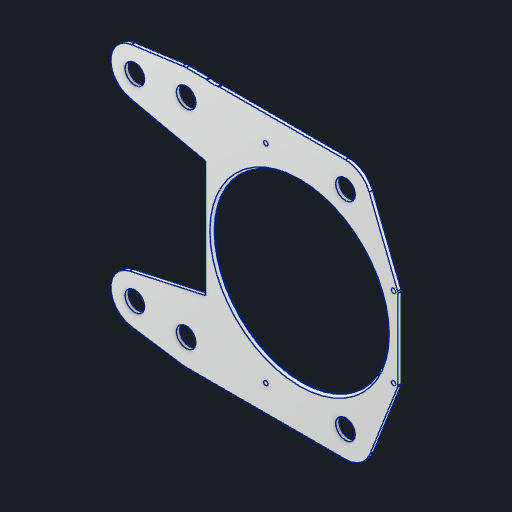
# Autodesk Inventor part: OUTK_002_ShotPlateReceptacle
Saved by Autodesk Inventor 2024.2 (Build 282272000, 272)
## iProperties
Created: 2024-11-24
Part Number: OUTK_002_ShotPlateReceptacle
Material: Aluminum 6061
Document SubType Name: Modeling
Designer: Bryan
Density: 2.7 g/cm^3
Appearance: Aluminum - Flat
Mass: 837.54 g
Surface Area: 1450.99 cm^2
Volume: 310.2 cm^3
Author: Bryan
Autodesk Inventor part; units mm, degrees
ref_plane "YZ Plane" through (0, 0, 0) normal (1, 0, 0) x (0, 1, 0)
ref_plane "XZ Plane" through (0, 0, 0) normal (0, 1, 0) x (-1, 0, 0)
ref_plane "XY Plane" through (0, 0, 0) normal (0, 0, 1) x (1, 0, 0)
sketch "Sketch1" plane through (0, 0, 0) normal (0, 0, 1) x (1, 0, 0)
  circle A0 centre (0, 142.875) radius 63.5 construction
  circle A1 centre (0, 142.875) radius 25.4 construction
  circle A2 centre (0, -142.875) radius 25.4 construction
  circle A3 centre (0, -142.875) radius 63.5 construction
  line L0 (0, 79.375) -> (0, 79.375) construction
  line L1 (0, -79.375) -> (0, -79.375) construction
  line L2 (0, 0) -> (229.6782, 0) construction
  line L3 (0, 142.875) -> (305.8782, 142.875) construction
  line L4 (305.8782, 142.875) -> (305.8782, -142.875) construction
  line L5 (305.8782, -142.875) -> (0, -142.875) construction
  circle A4 centre (229.6782, 0) radius 127 construction
  circle A5 centre (0, 142.875) radius 14.2875
  circle A6 centre (0, -142.875) radius 14.2875
  circle A7 centre (0, 142.875) radius 34.925 construction
  circle A8 centre (0, -142.875) radius 34.925 construction
  circle A9 centre (74.585, -150.8125) radius 22.225 construction
  circle A10 centre (74.585, -150.8125) radius 33.3375 construction
  circle A11 centre (74.585, -150.8125) radius 11.1125 construction
  line L6 (74.585, -139.7) -> (74.585, -128.5875) construction
  line L7 (74.585, -117.475) -> (74.585, -128.5875) construction
  circle A12 centre (305.8782, -150.8125) radius 33.3375 construction
  circle A13 centre (305.8782, -150.8125) radius 14.2875
  circle A14 centre (375.7282, 58.0572) radius 6.35 construction
  circle A15 centre (375.7282, -58.0572) radius 6.35 construction
  line L8 (305.8782, 150.8125) -> (375.7282, 58.0572) construction
  line L9 (375.7282, 58.0572) -> (375.7282, -58.0572) construction
  line L10 (375.7282, -58.0572) -> (305.8782, -150.8125) construction
  line L11 (-117.6668, 84.5312) -> (102.6782, 84.5312) construction
  line L12 (102.6782, 84.5312) -> (102.6782, -84.5312) construction
  line L13 (102.6782, -84.5312) -> (-117.6668, -84.5312) construction
  line L14 (-117.6668, -84.5312) -> (-117.6668, 84.5312) construction
  line L15 (0, 142.875) -> (0, 84.5312) construction
  line L16 (0, -84.5312) -> (0, -142.875) construction
  circle A16 centre (74.585, -150.8125) radius 14.2875
  line L17 (74.585, -117.475) -> (305.8782, -117.475) construction
  circle A17 centre (74.585, 0) radius 127 construction
  circle A18 centre (0, 0) radius 127 construction
  circle A19 centre (0, 142.875) radius 6.35 construction
  circle A20 centre (74.585, 150.8125) radius 33.3375 construction
  circle A21 centre (305.8782, 150.8125) radius 33.3375 construction
  circle A22 centre (305.8782, 150.8125) radius 14.2875
  circle A23 centre (74.585, 150.8125) radius 14.2875
  circle A24 centre (74.585, 150.8125) radius 37.1475 construction
  circle A25 centre (305.8782, 150.8125) radius 37.1475 construction
  circle A26 centre (305.8782, -150.8125) radius 38.1 construction
  circle A27 centre (74.585, -150.8125) radius 38.1 construction
  line L18 (-4.7233, 177.4791) -> (69.5611, 187.6187)
  line L19 (74.585, 187.96) -> (305.8782, 187.96)
  line L20 (340.4169, 164.488) -> (381.6323, 60.3949)
  line L21 (382.0782, 58.0572) -> (382.0782, -58.0572)
  line L22 (68.953, -188.4939) -> (-5.1627, -177.4163)
  line L23 (221.4945, -245.7989) -> (238.8691, -293.5353) construction
  line L24 (238.8691, -293.5353) -> (382.0782, -241.4114) construction
  line L25 (382.0782, -241.4114) -> (364.7036, -193.675) construction
  line L26 (364.7036, -193.675) -> (221.4945, -245.7989) construction
  line L27 (-7.5024, -108.7653) -> (102.6782, -84.5312)
  line L28 (-7.5024, 108.7653) -> (102.6782, 84.5312)
  line L29 (102.6782, 84.5312) -> (102.6782, -84.5312)
  circle A28 centre (239.2032, 0) radius 127
  line L30 (102.6782, 0) -> (112.2032, 0)
  line L31 (375.7282, 0) -> (366.2032, 0)
  circle A29 centre (221.4945, -245.7989) radius 3.2512 construction
  circle A30 centre (269.2308, -228.4242) radius 3.2512 construction
  circle A31 centre (316.9672, -211.0496) radius 3.2512 construction
  circle A32 centre (364.7036, -193.675) radius 3.2512 construction
  circle A33 centre (238.8691, -293.5353) radius 3.2512 construction
  circle A34 centre (286.6055, -276.1606) radius 3.2512 construction
  circle A35 centre (334.3418, -258.786) radius 3.2512 construction
  circle A36 centre (382.0782, -241.4114) radius 3.2512 construction
  line L32 (74.585, -188.9125) -> (305.8782, -188.9125)
  line L33 (381.652, -60.3445) -> (341.4207, -164.5364)
  arc A37 (-4.7233, 177.4791) -> (-7.5024, 108.7653) centre (0, 142.875) ccw
  arc A38 (74.585, 187.96) -> (69.5611, 187.6187) centre (74.585, 150.8125) ccw
  arc A39 (340.4169, 164.488) -> (305.8782, 187.96) centre (305.8782, 150.8125) ccw
  arc A40 (382.0782, 58.0572) -> (381.6323, 60.3949) centre (375.7282, 58.0572) ccw
  arc A41 (381.652, -60.3445) -> (382.0782, -58.0572) centre (375.7282, -58.0572) ccw
  arc A42 (305.8782, -188.9125) -> (341.4207, -164.5364) centre (305.8782, -150.8125) ccw
  arc A43 (68.953, -188.4939) -> (74.585, -188.9125) centre (74.585, -150.8125) ccw
  arc A44 (-7.5024, -108.7653) -> (-5.1627, -177.4163) centre (0, -142.875) ccw
  circle A45 centre (375.7282, 58.0572) radius 3.2512
  circle A46 centre (375.7282, -58.0572) radius 3.2512
  circle A47 centre (190.2316, 150.8125) radius 3.2512
  line L34 (74.585, 150.8125) -> (190.2316, 150.8125) construction
  line L35 (190.2316, 150.8125) -> (305.8782, 150.8125) construction
  circle A48 centre (190.2316, -150.8125) radius 3.2512
  point P0 (0, 117.475)
  point P1 (0, -117.475)
  point P2 (305.8782, 0)
  point P3 (229.6782, -127)
  point P4 (229.6782, -127)
  point P5 (356.6782, 0)
  point P6 (0, 127)
  point P7 (0, 117.475)
  point P8 (0, 136.525)
  dimension "d1" = 50.8
  dimension "d16" = 44.45
  dimension "d20" = 22.225
  dimension "d33" = 12.7
  dimension "d0" = 127
  dimension "d3" = 285.75
  dimension "d4" = 254
  dimension "d6" = 158.75
  dimension "d7" = 234.95
  dimension "d11" = 28.575
  dimension "d12" = 28.575
  dimension "d13" = 69.85
  dimension "d14" = 69.85
  dimension "d19" = 76.2
  dimension "d24" = 28.575
  dimension "d26" = 12.7
  dimension "d27" = 12.7
  dimension "d28" = 19.05
  dimension "d29" = 220.345
  dimension "d30" = 169.0624
  dimension "d31" = 9.525
  dimension "d32" = 75.0062
  dimension "d34" = 9.525
  dimension "d35" = 19.05
  dimension "d37" = 3.81
  dimension "d38" = 3.81
  dimension "d39" = 4.7625
  dimension "d40" = 4.7625
  dimension "d43" = 20
  dimension "d44" = 6.5024
  dimension "d47" = 50.8
  dimension "d50" = 50.8
  dimension "d53" = 50.8
  dimension "d56" = 6.5024
  dimension "d57" = 6.5024
  dimension "d58" = 6.5024
  dimension "d108" = 231.2932
  constraints: 72 end point, 41 centre point, 41 point on circle, 24 tangent, 21 coincident, 16 vertical alignment, 11 horizontal, 7 perpendicular, 7 point on line, 6 concentric, 6 equal length, 6 symmetric about line, 4 equal radius, 4 vertical, 3 horizontal alignment, 3 midpoint, 2 parallel, 41 other
  measures "d0" diameter of A0
  measures "d3" distance between parallel lines of L5 L3
  measures "d4" diameter of A4
  measures "d6" distance of L1.start L0.start
  measures "d7" distance of point (0, -117.475) point (0, 117.475)
  measures "d11" diameter of A5
  measures "d12" diameter of A6
  measures "d13" diameter of A7
  measures "d14" diameter of A8
  measures "d19" distance of point (305.878, 0) L2.end
  measures "d24" diameter of A13
  measures "d26" diameter of A14
  measures "d27" diameter of A15
  measures "d28" distance from line of L9 point (356.678, 0)
  measures "d29" distance of L12.end L13.end
  measures "d30" distance of L11.end L12.end
  measures "d31" distance from line of L17 A4.start
  measures "d32" distance of point (74.585, -150.812) point (0, -142.875)
  measures "d34" distance of point (0, 117.475) point (0, 127)
  measures "d35" distance of point (0, 117.475) point (0, 136.525)
  measures "d37" radial gap between concentric circles of A20 A24
  measures "d38" radial gap between concentric circles of A21 A25
  measures "d43" angle of L26 L5
  measures "d44" diameter of A29
  measures "d47" distance of A29.centre A30.centre
  measures "d50" distance of A29.centre A33.centre
  measures "d53" distance from line of L25.end L5
  measures "d56" diameter of A45
  measures "d57" diameter of A46
  measures "d58" diameter of A47
  measures "d108" distance of L8.start A23.centre
extrude "Extrusion1" add sketch "Sketch1" along normal mid plane 4.7625
sketch "Sketch2" plane through (0, 0, -2.3813) normal (0, 0, -1) x (-1, 0, 0)
  line L0 (7.5024, -108.7653) -> (-102.6782, -84.5312) projected
  line L1 (-102.6782, -84.5312) -> (-102.6782, 84.5312) projected
  line L2 (-102.6782, 84.5312) -> (7.5024, 108.7653) projected
  arc A0 (7.5024, 108.7653) -> (4.7233, 177.4791) centre (0, 142.875) ccw projected
  line L3 (4.7233, 177.4791) -> (-69.5611, 187.6187) projected
  arc A1 (-69.5611, 187.6187) -> (-74.585, 187.96) centre (-74.585, 150.8125) ccw projected
  line L4 (-74.585, 187.96) -> (-305.8782, 187.96) projected
  arc A2 (-305.8782, 187.96) -> (-340.4169, 164.488) centre (-305.8782, 150.8125) ccw projected
  line L5 (-340.4169, 164.488) -> (-381.6323, 60.3949) projected
  arc A3 (-381.6323, 60.3949) -> (-382.0782, 58.0572) centre (-375.7282, 58.0572) ccw projected
  line L6 (-382.0782, 58.0572) -> (-382.0782, -58.0572) projected
  arc A4 (-382.0782, -58.0572) -> (-381.652, -60.3445) centre (-375.7282, -58.0572) ccw projected
  line L7 (-381.652, -60.3445) -> (-341.4207, -164.5364) projected
  arc A5 (-341.4207, -164.5364) -> (-305.8782, -188.9125) centre (-305.8782, -150.8125) ccw projected
  line L8 (-305.8782, -188.9125) -> (-74.585, -188.9125) projected
  arc A6 (-74.585, -188.9125) -> (-68.953, -188.4939) centre (-74.585, -150.8125) ccw projected
  line L9 (-68.953, -188.4939) -> (5.1627, -177.4163) projected
  arc A7 (5.1627, -177.4163) -> (7.5024, -108.7653) centre (0, -142.875) ccw projected
  circle A8 centre (-239.2032, 0) radius 127 projected
  circle A9 centre (-74.585, -150.8125) radius 14.2875 projected
  circle A10 centre (-74.585, 150.8125) radius 14.2875 projected
  circle A11 centre (-190.2316, 150.8125) radius 3.2512 projected
  circle A12 centre (-190.2316, -150.8125) radius 3.2512 projected
  circle A13 centre (-375.7282, -58.0572) radius 3.2512 projected
  circle A14 centre (-375.7282, 58.0572) radius 3.2512 projected
  circle A15 centre (-305.8782, 150.8125) radius 14.2875 projected
  circle A16 centre (-305.8782, -150.8125) radius 14.2875 projected
  circle A17 centre (0, -142.875) radius 14.2875 projected
  circle A18 centre (0, 142.875) radius 14.2875 projected
  line L10 (-107.4407, -88.36) -> (6.4793, -113.4166)
  arc A19 (4.4587, -172.7061) -> (6.4793, -113.4166) centre (0, -142.875) ccw
  line L11 (4.4587, -172.7061) -> (-69.657, -183.7838)
  arc A20 (-74.585, -184.15) -> (-69.657, -183.7838) centre (-74.585, -150.8125) ccw
  line L12 (-74.585, -184.15) -> (-305.8782, -184.15)
  arc A21 (-336.9779, -162.8209) -> (-305.8782, -184.15) centre (-305.8782, -150.8125) ccw
  line L13 (-336.9779, -162.8209) -> (-377.2092, -58.6291)
  arc A22 (-377.3157, -58.0572) -> (-377.2092, -58.6291) centre (-375.7282, -58.0572) ccw
  line L14 (-377.3157, -58.0572) -> (-377.3157, 58.0572)
  arc A23 (-377.2042, 58.6416) -> (-377.3157, 58.0572) centre (-375.7282, 58.0572) ccw
  line L15 (-377.2042, 58.6416) -> (-335.9888, 162.7347)
  arc A24 (-305.8782, 183.1975) -> (-335.9888, 162.7347) centre (-305.8782, 150.8125) ccw
  line L16 (-305.8782, 183.1975) -> (-74.585, 183.1975)
  arc A25 (-70.2052, 182.9) -> (-74.585, 183.1975) centre (-74.585, 150.8125) ccw
  line L17 (-70.2052, 182.9) -> (4.0793, 172.7604)
  arc A26 (6.4793, 113.4166) -> (4.0793, 172.7604) centre (0, 142.875) ccw
  line L18 (6.4793, 113.4166) -> (-107.4407, 88.36)
  line L19 (-107.4407, 88.36) -> (-107.4407, -88.36)
  circle A27 centre (-239.2032, 0) radius 133.35
  circle A28 centre (-74.585, 150.8125) radius 19.05
  circle A29 centre (0, 142.875) radius 19.05
  circle A30 centre (-190.2316, 150.8125) radius 8.0137
  circle A31 centre (-305.8782, 150.8125) radius 19.05
  circle A32 centre (-375.7282, 58.0572) radius 8.0137
  circle A33 centre (-375.7282, -58.0572) radius 8.0137
  circle A34 centre (-305.8782, -150.8125) radius 19.05
  circle A35 centre (-190.2316, -150.8125) radius 8.0137
  circle A36 centre (-74.585, -150.8125) radius 19.05
  circle A37 centre (0, -142.875) radius 19.05
  line L20 (0, -142.875) -> (-74.585, -150.8125)
  line L21 (-74.585, -150.8125) -> (-71.7613, -188.8077)
  line L22 (-74.585, -150.8125) -> (-102.6782, -84.5312)
  line L23 (-74.585, -150.8125) -> (-190.2316, -150.8125)
  line L24 (-190.2316, -150.8125) -> (-190.2316, -188.9125)
  line L25 (-190.2316, -150.8125) -> (-305.8782, -150.8125)
  line L26 (-305.8782, -150.8125) -> (-327.4274, -182.233)
  line L27 (-102.6782, -84.5312) -> (-239.2032, 0)
  line L28 (-239.2032, 0) -> (-190.2316, -150.8125)
  line L29 (-305.8782, -150.8125) -> (-239.2032, 0)
  line L30 (-239.2032, 0) -> (-375.7282, -58.0572)
  line L31 (-239.2032, 0) -> (-375.7282, 58.0572)
  line L32 (-375.7282, 58.0572) -> (-305.8782, 150.8125)
  line L33 (-305.8782, 150.8125) -> (-190.2316, 150.8125)
  line L34 (-190.2316, 150.8125) -> (-74.585, 150.8125)
  line L35 (-74.585, 150.8125) -> (0, 142.875)
  line L36 (-102.6782, -84.5312) -> (-190.2316, -150.8125)
  line L37 (-305.8782, -150.8125) -> (-375.7282, -58.0572)
  line L38 (-102.6782, 84.5312) -> (-74.585, 150.8125)
  line L39 (-102.6782, 84.5312) -> (-190.2316, 150.8125)
  line L40 (-102.6782, 84.5312) -> (-239.2032, 0)
  line L41 (-239.2032, 0) -> (-190.2316, 150.8125)
  line L42 (-239.2032, 0) -> (-305.8782, 150.8125)
  line L43 (-4.7625, -138.5924) -> (-75.089, -146.0767)
  line L44 (-68.936, -151.9364) -> (-99.5574, -79.6902)
  line L45 (0, -142.875) -> (0, -111.9915)
  line L46 (-4.7625, -110.944) -> (-4.7625, -138.5924)
  line L47 (0, 142.875) -> (0, 111.9915)
  line L48 (-99.5574, 79.6902) -> (-68.936, 151.9364)
  line L49 (-108.3272, 83.4073) -> (-77.7058, 155.6535)
  line L50 (-190.2316, 146.05) -> (-74.585, 146.05)
  line L51 (-98.0687, 87.0149) -> (-189.092, 155.923)
  line L52 (-105.1853, 88.5804) -> (-241.7103, 4.0492)
  line L53 (-103.8179, 79.4207) -> (-194.8411, 148.3288)
  line L54 (-235.7016, -4.6369) -> (-184.6739, 152.5077)
  line L55 (-244.761, -1.6952) -> (-193.7332, 155.4494)
  line L56 (-305.8782, 146.05) -> (-190.2316, 146.05)
  line L57 (-233.5511, -1.0064) -> (-302.8187, 155.6703)
  line L58 (-242.2627, -4.8578) -> (-311.5303, 151.8189)
  line L59 (-300.8665, 149.5508) -> (-368.2605, 60.0568)
  line L60 (-368.2605, 60.0568) -> (-236.9729, 4.2268)
  line L61 (-240.7003, -4.5386) -> (-383.1959, 56.0576)
  line L62 (-383.1959, 56.0576) -> (-308.4753, 155.2807)
  line L63 (-240.7003, 4.5386) -> (-383.1959, -56.0576)
  line L64 (-383.1959, -56.0576) -> (-308.4753, -155.2807)
  line L65 (-236.9729, -4.2268) -> (-368.2605, -60.0568)
  line L66 (-368.2605, -60.0568) -> (-300.8665, -149.5508)
  line L67 (-311.5303, -151.8189) -> (-242.2627, 4.8578)
  line L68 (-244.761, 1.6952) -> (-193.7332, -155.4494)
  line L69 (-235.7016, 4.6369) -> (-184.6739, -152.5077)
  line L70 (-302.8187, -155.6703) -> (-233.5511, 1.0064)
  line L71 (-105.1853, -88.5804) -> (-241.7103, -4.0492)
  line L72 (-100.1711, -80.482) -> (-236.6961, 4.0492)
  line L73 (-100.1711, 80.482) -> (-236.6961, -4.0492)
  line L74 (-77.7058, -155.6535) -> (-108.3272, -83.4073)
  line L75 (-105.5995, -80.7694) -> (-196.6227, -149.6775)
  line L76 (-98.0687, -87.0149) -> (-189.092, -155.923)
  line L77 (-74.585, -146.05) -> (-190.2316, -146.05)
  line L78 (-190.2316, -146.05) -> (-305.8782, -146.05)
  line L79 (-75.089, 146.0767) -> (-4.7625, 138.5924)
  line L80 (-4.7625, 138.5924) -> (-4.7625, 110.944)
  arc A38 (-377.3157, -6.35) -> (-372.4074, -6.2352) centre (-374.8602, -6.35) ccw
  arc A39 (-372.4074, 6.2352) -> (-377.3157, 6.35) centre (-374.8602, 6.35) ccw
  line L81 (-239.2032, 0) -> (-366.2032, 0)
  point P0 (0, 0)
  dimension "d59" = 4.7625
  dimension "d60" = 6.35
  dimension "d61" = 4.7625
  dimension "d62" = 4.7625
  dimension "d63" = 4.7625
  dimension "d64" = 4.7625
  dimension "d65" = 4.7625
  dimension "d66" = 4.7625
  dimension "d67" = 4.7625
  dimension "d68" = 4.7625
  dimension "d69" = 4.7625
  dimension "d70" = 4.7625
  dimension "d71" = 4.7625
  dimension "d72" = 4.7625
  dimension "d73" = 4.7625
  dimension "d75" = 4.7625
  dimension "d76" = 4.7625
  dimension "d77" = 4.7625
  dimension "d78" = 4.7625
  dimension "d79" = 4.7625
  dimension "d80" = 4.7625
  dimension "d81" = 4.7625
  dimension "d82" = 4.7625
  dimension "d83" = 4.7625
  dimension "d84" = 4.7625
  dimension "d85" = 4.7625
  dimension "d86" = 4.7625
  dimension "d87" = 4.7625
  dimension "d88" = 4.7625
  dimension "d89" = 4.7625
  dimension "d90" = 4.7625
  dimension "d91" = 4.7625
  dimension "d92" = 4.7625
  dimension "d93" = 4.7625
  dimension "d94" = 4.7625
  dimension "d95" = 4.7625
  dimension "d96" = 4.7625
  dimension "d97" = 4.7625
  dimension "d98" = 4.7625
  dimension "d99" = 4.7625
  dimension "d100" = 4.7625
  dimension "d101" = 4.7625
  dimension "d102" = 4.7625
  dimension "d103" = 4.7625
  dimension "d104" = 12.7
  constraints: 144 end point, 25 parallel, 24 point on circle, 21 centre point, 6 point on line, 5 horizontal, 4 tangent, 2 vertical, 1 horizontal alignment, 1 midpoint, 1 symmetric about line, 22 other
  measures "d59" distance between parallel lines of L0 L10
  measures "d61" radial gap between concentric circles of A10 A28
  measures "d62" radial gap between concentric circles of A18 A29
  measures "d63" radial gap between concentric circles of A11 A30
  measures "d64" radial gap between concentric circles of A15 A31
  measures "d65" radial gap between concentric circles of A14 A32
  measures "d66" radial gap between concentric circles of A13 A33
  measures "d67" radial gap between concentric circles of A16 A34
  measures "d68" radial gap between concentric circles of A12 A35
  measures "d69" radial gap between concentric circles of A9 A36
  measures "d70" radial gap between concentric circles of A17 A37
  measures "d71" distance between parallel lines of L20 L43
  measures "d72" distance between parallel lines of L22 L44
  measures "d73" distance between parallel lines of L45 L46
  measures "d75" distance between parallel lines of L38 L48
  measures "d76" distance between parallel lines of L38 L49
  measures "d77" distance between parallel lines of L34 L50
  measures "d78" distance between parallel lines of L39 L51
  measures "d79" distance between parallel lines of L40 L52
  measures "d80" distance between parallel lines of L39 L53
  measures "d81" distance between parallel lines of L41 L54
  measures "d82" distance between parallel lines of L41 L55
  measures "d83" distance between parallel lines of L33 L56
  measures "d84" distance between parallel lines of L42 L57
  measures "d85" distance between parallel lines of L42 L58
  measures "d86" distance between parallel lines of L32 L59
  measures "d87" distance between parallel lines of L31 L61
  measures "d88" distance between parallel lines of L30 L63
  measures "d89" distance between parallel lines of L30 L65
  measures "d90" distance between parallel lines of L29 L67
  measures "d91" distance between parallel lines of L28 L68
  measures "d92" distance between parallel lines of L28 L69
  measures "d93" distance between parallel lines of L29 L70
  measures "d94" distance between parallel lines of L27 L71
  measures "d95" distance between parallel lines of L27 L72
  measures "d96" distance between parallel lines of L40 L73
  measures "d97" distance between parallel lines of L22 L74
  measures "d98" distance between parallel lines of L36 L75
  measures "d99" distance between parallel lines of L36 L76
  measures "d100" distance between parallel lines of L23 L77
  measures "d101" distance between parallel lines of L25 L78
  measures "d102" distance between parallel lines of L35 L79
  measures "d103" distance between parallel lines of L47 L80
  measures "d104" distance of A39.centre A38.centre
chamfer "Chamfer1" distance 3.175 distance2 3.175 1 edges at (112.2032, 0, 2.3813) measured on face at (190.101, -177.2883, 2.3812)
sketch "Sketch3" plane through (0, 0, 2.3813) normal (0, 0, 1) x (1, 0, 0)
  line L0 (305.8782, 187.96) -> (74.585, 187.96) projected
  arc A0 (104.1636, 187.96) -> (121.7761, 187.96) centre (112.9698, 216.6384) ccw
  circle A1 centre (117.1583, 219.0822) radius 4 projected
  circle A2 centre (112.9698, 216.6384) radius 2.0193 projected
  point P0 (0, 0)
  dimension "d109" = 30
  constraints: 2 point on circle, 2 point on line, 1 centre point, 1 coincident
  measures "d109" radius of A0
extrude "Extrusion2" cut sketch "Sketch3" against normal blind 25.4 contours A0 L0
fillet "Fillet1" radius 6.35 2 edges at (104.1636, 187.96, 0) (121.7761, 187.96, 0)
body "Solid1"
